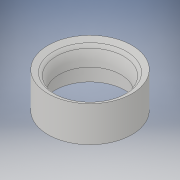
# Autodesk Inventor part: Graphite
Saved by Autodesk Inventor 2017 (Build 210142000, 142)
## iProperties
Created: 2016-07-19
Part Number: Graphite
Material: Generic
Document SubType Name: Modeling
Designer: Bill
Density: 1 g/cm^3
Appearance: Default
Author: Bill
Autodesk Inventor part; units mm, degrees
ref_plane "YZ Plane" through (0, 0, 0) normal (1, 0, 0) x (0, 1, 0)
ref_plane "XZ Plane" through (0, 0, 0) normal (0, 1, 0) x (-1, 0, 0)
ref_plane "XY Plane" through (0, 0, 0) normal (0, 0, 1) x (1, 0, 0)
sketch "Sketch1" plane through (0, 0, 0) normal (0, 0, 1) x (1, 0, 0)
  line L0 (-38.9636, -24.3633) -> (-32.6136, -24.3633)
  line L1 (-32.6136, -24.3633) -> (-28.702, -9.765)
  line L2 (-38.9636, -24.3633) -> (-38.9636, 8.6567)
  line L3 (-38.9636, 8.6567) -> (-33.8941, 6.2928)
  line L4 (-38.9636, 8.6567) -> (-32.2265, 8.6567) construction
  arc A0 (-28.702, -9.765) -> (-31.3296, 3.6475) centre (-49.4557, -6.8672) ccw
  arc A1 (-31.3296, 3.6475) -> (-33.8941, 6.2928) centre (-36.5924, 1.1112) ccw
  line L5 (0, -30.9673) -> (0, 15.2607) projected
  point P0 (0, 0)
  dimension "d0" = 105
  dimension "d1" = 6.35
  dimension "d2" = 32.6136
  dimension "d3" = 28.702
  dimension "d4" = 33.02
  dimension "d5" = 25
  dimension "d6" = 5.842
  dimension "d7" = 20.955
  constraints: 10 end point, 4 point on circle, 2 centre point, 2 horizontal, 1 vertical
  measures "d0" angle of L0 L1
  measures "d1" distance of L0.start L0.end
  measures "d2" horizontal distance of point (0, 0) L0.end
  measures "d3" horizontal distance of point (0, 0) L1.end
  measures "d4" distance of L0.start L2.end
  measures "d5" angle of L4 L3
  measures "d6" radius of A1
  measures "d7" radius of A0
revolve "Revolution1" add sketch "Sketch1" angle 360 about axis through (0, -10, 0) along (0, 1, 0)
body "Solid1"
